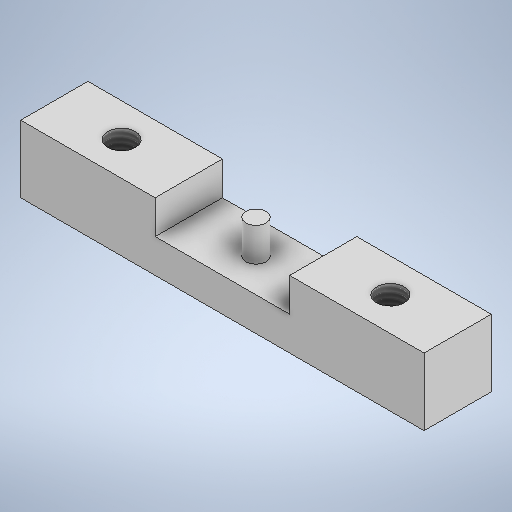
# Autodesk Inventor part: środek
Saved by Autodesk Inventor 2025.2 (Build 292293000, 293)
## iProperties
Created: 2026-05-07
Part Number: środek
Material: Ogólny
Document SubType Name: Modeling
Designer: muszy
Density: 1 g/cm^3
Appearance: Domyślna
Author: muszy
Autodesk Inventor part; units mm, degrees
ref_plane "YZ Plane" through (0, 0, 0) normal (1, 0, 0) x (0, 1, 0)
ref_plane "XZ Plane" through (0, 0, 0) normal (0, 1, 0) x (-1, 0, 0)
ref_plane "XY Plane" through (0, 0, 0) normal (0, 0, 1) x (1, 0, 0)
sketch "Szkic1" plane through (0, 0, 0) normal (0, 0, 1) x (1, 0, 0)
  point P0 (0, 0)
sketch "Szkic2" plane through (0, 0, 0) normal (0, 1, 0) x (-1, 0, 0)
  line L0 (30, 5) -> (-30, 5)
  line L1 (-30, 5) -> (-30, -5)
  line L2 (-30, -5) -> (30, -5)
  line L3 (30, -5) -> (30, 5)
  line L4 (13.3205, 0) -> (-15.9073, 0) construction
  line L5 (0, 22.8583) -> (0, -40.0607) construction
  point P0 (0, 0)
  dimension "d0" = 10
  dimension "d1" = 60
  constraints: 12 end point, 2 horizontal, 2 parallel, 2 perpendicular, 1 vertical, 2 other
  measures "d0" distance between parallel lines of L2 L0
  measures "d1" distance between parallel lines of L1 L3
extrude "Wyciągnięcie proste1" add sketch "Szkic2" along normal blind 5
sketch "Szkic3" plane through (0, 5, 0) normal (0, 1, 0) x (1, 0, 0)
  line L0 (-30, 5) -> (-30, -5) projected
  line L1 (30, 5) -> (-30, 5) projected
  line L2 (-30, -5) -> (-10, -5)
  line L3 (-10, -5) -> (-10, 5)
  line L4 (-10, 5) -> (-30, 5)
  line L5 (-30, 5) -> (-30, -5)
  line L6 (30, -5) -> (10, -5)
  line L7 (10, -5) -> (10, 5)
  line L8 (10, 5) -> (30, 5)
  line L9 (30, 5) -> (30, -5)
  line L10 (0, 41.547) -> (0, -40.407) construction
  circle A0 centre (0, 0) radius 1.5
  dimension "d4" = 20
  dimension "d5" = 20
  dimension "d6" = 3
  constraints: 18 end point, 4 parallel, 3 point on line, 2 horizontal, 2 perpendicular, 1 centre point, 1 coincident, 1 vertical, 1 other
  measures "d4" distance between parallel lines of L0 L3
  measures "d5" distance between parallel lines of L9 L7
  measures "d6" diameter of A0
extrude "Wyciągnięcie proste2" add sketch "Szkic3" along normal blind 5
sketch "Szkic4" plane through (0, 10, 0) normal (0, 1, 0) x (1, 0, 0)
  line L0 (0, 14.0263) -> (0, -15.9036) construction
  line L1 (-30, 5) -> (-30, -5) projected
  point P0 (0, 0)
  point P1 (-20, 0)
  point P2 (20, 0)
  dimension "d9" = 10
  constraints: 2 end point, 1 symmetric about line, 1 vertical
  measures "d9" distance from line of point (-20, 0) L1
hole "Otwór1" at (-20, 10, 0) at (20, 10, 0) direction (0, -1, 0) diameter 4.134 depth 5 tip angle 118 thread size "M5x0.8" class "6H" standard "ISO Metric profile"
